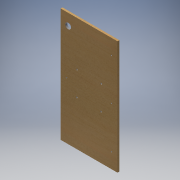
# Autodesk Inventor part: toit
Saved by Autodesk Inventor 2019 (Build 230136000, 136)
## iProperties
Created: 2018-04-02
Part Number: toit
Material: Générique
Document SubType Name: Modeling
Designer: franc
Density: 1 g/cm^3
Appearance: Par défaut
Author: franc
Autodesk Inventor part; units mm, degrees
ref_plane "YZ Plane" through (0, 0, 0) normal (1, 0, 0) x (0, 1, 0)
ref_plane "XZ Plane" through (0, 0, 0) normal (0, 1, 0) x (-1, 0, 0)
ref_plane "XY Plane" through (0, 0, 0) normal (0, 0, 1) x (1, 0, 0)
sketch "Esquisse1" plane through (0, 0, 0) normal (0, 1, 0) x (-1, 0, 0)
  line L0 (110.1985, 107.2202) -> (-39.8015, 107.2202)
  line L1 (-39.8015, 107.2202) -> (-39.8015, -192.7798)
  line L2 (-39.8015, -192.7798) -> (110.1985, -192.7798)
  line L3 (110.1985, -192.7798) -> (110.1985, 107.2202)
  point P0 (0, 0)
  dimension "d0" = 300
  dimension "d1" = 150
  constraints: 8 end point, 2 parallel, 1 horizontal, 1 perpendicular
  measures "d0" distance of L2.end L0.start
  measures "d1" distance of L0.start L0.end
extrude "Extrusion1" add sketch "Esquisse1" along normal blind 5
sketch "Esquisse2" plane through (0, 0, 0) normal (0, -1, 0) x (1, 0, 0)
  circle A0 centre (-94.1985, -42.7798) radius 1.5
  circle A1 centre (23.8015, -42.7798) radius 1.5
  circle A2 centre (23.8015, 67.2202) radius 1.5
  circle A3 centre (23.8015, -152.7798) radius 1.5
  line L0 (-110.1985, -192.7798) -> (-110.1985, 107.2202) projected
  line L1 (39.8015, -192.7798) -> (-110.1985, -192.7798) projected
  line L2 (39.8015, 107.2202) -> (39.8015, -192.7798) projected
  line L3 (-110.1985, 107.2202) -> (39.8015, 107.2202) projected
  point P0 (0, 0)
  dimension "d4" = 16
  dimension "d5" = 150
  dimension "d6" = 16
  dimension "d7" = 16
  dimension "d8" = 16
  dimension "d9" = 40
  dimension "d10" = 150
  dimension "d11" = 40
  constraints: 4 centre point
  measures "d4" distance from line of L0 A0.centre
  measures "d5" distance from line of L1 A0.centre
  measures "d6" distance from line of L2 A2.centre
  measures "d7" distance from line of L2 A1.centre
  measures "d8" distance from line of L2 A3.centre
  measures "d9" distance from line of L1 A3.centre
  measures "d10" distance from line of L1 A1.centre
  measures "d11" distance from line of L3 A2.centre
extrude "Extrusion2" cut sketch "Esquisse2" against normal through all contours A0 | A1 | A2 | A3
sketch "Esquisse6" plane through (0, 0, 0) normal (0, -1, 0) x (1, 0, 0)
  circle A0 centre (-90.1985, 77.2202) radius 7.5
  line L0 (-110.1985, 107.2202) -> (39.8015, 107.2202) projected
  line L1 (-110.1985, -192.7798) -> (-110.1985, 107.2202) projected
  point P0 (0, 0)
  dimension "d32" = 15
  dimension "d33" = 30
  dimension "d34" = 20
  constraints: 1 centre point
  measures "d32" diameter of A0
  measures "d33" distance from line of L0 A0.centre
  measures "d34" distance from line of L1 A0.centre
extrude "Extrusion6" cut sketch "Esquisse6" against normal up to next
sketch "Esquisse8" plane through (0, 5, 0) normal (0, 1, 0) x (1, 0, 0)
  circle A0 centre (-67.021, 10.6032) radius 2
  circle A1 centre (-3.0219, 10.9574) radius 2
  circle A2 centre (-3.3761, 74.9564) radius 2
  circle A3 centre (-67.3752, 74.6022) radius 2
  point P0 (0, 0)
  constraints: 4 centre point, 8 other
extrude "Extrusion8" cut sketch "Esquisse8" against normal through all
